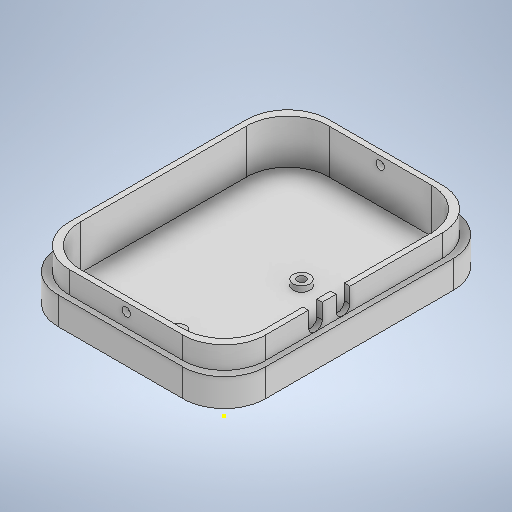
# Autodesk Inventor part: reduced_tortoise_3_base
Saved by Autodesk Inventor 2025.1 (Build 291241000, 241)
## iProperties
Created: 2025-04-15
Part Number: reduced_tortoise_3_base
Material: Generic
Document SubType Name: Modeling
Designer: Ian Ching
Density: 1 g/cm^3
Appearance: Default
Author: Ian Ching
Autodesk Inventor part; units mm, degrees
ref_plane "YZ Plane" through (0, 0, 0) normal (1, 0, 0) x (0, 1, 0)
ref_plane "XZ Plane" through (0, 0, 0) normal (0, 1, 0) x (-1, 0, 0)
ref_plane "XY Plane" through (0, 0, 0) normal (0, 0, 1) x (1, 0, 0)
sketch "Sketch1" plane through (0, 0, 0) normal (0, 1, 0) x (-1, 0, 0)
  line L0 (0, 0) -> (75, 0)
  line L1 (75, 0) -> (75, -98)
  line L2 (75, -98) -> (0, -98)
  line L3 (0, -98) -> (0, 0)
  dimension "d0" = 75
  dimension "d1" = 98
  constraints: 8 end point, 2 parallel, 1 horizontal, 1 perpendicular
  measures "d0" distance of L1.end L2.end
  measures "d1" distance of L0.end L1.end
extrude "Extrusion1" add sketch "Sketch1" along normal blind 2
sketch "Sketch2" plane through (0, 2, 0) normal (0, 1, 0) x (1, 0, 0)
  line L0 (-75, 0) -> (0, 0)
  line L1 (0, 0) -> (0, 98)
  line L2 (0, 98) -> (-75, 98)
  line L3 (-75, 98) -> (-75, 0)
  line L4 (-73, 2) -> (-2, 2)
  line L5 (-2, 2) -> (-2, 96)
  line L6 (-2, 96) -> (-73, 96)
  line L7 (-73, 96) -> (-73, 2)
  line L8 (-37.5, 2) -> (-37.5, 96)
  line L9 (-37.5, 0) -> (-37.5, 98)
  line L10 (-75, 0) -> (0, 0) projected
  line L11 (-37.5, 0) -> (-37.5, 98)
  line L12 (0, 98) -> (-75, 98) projected
  point P0 (-37.5, 49)
  dimension "d4" = 75
  dimension "d5" = 98
  dimension "d6" = 71
  dimension "d7" = 94
  constraints: 22 end point, 9 midpoint, 4 parallel, 2 horizontal, 2 perpendicular
  measures "d4" distance of L2.end L1.end
  measures "d5" distance of L1.end L0.end
  measures "d6" distance of L6.end L5.end
  measures "d7" distance of L5.end L4.end
extrude "Extrusion2" add sketch "Sketch2" along normal blind 8 contours L3 L2 L9 L6 L7 L4 L0 | L9 L4 L5 L6 L2 L1 L0
sketch "Sketch5" plane through (0, 2, 0) normal (0, 1, 0) x (1, 0, 0)
  line L0 (-2, 2) -> (-73, 2) projected
  line L1 (-73, 96) -> (-2, 96) projected
  line L2 (-2, 2) -> (-73, 2)
  line L3 (-73, 2) -> (-73, 96)
  line L4 (-73, 96) -> (-2, 96)
  line L5 (-2, 96) -> (-2, 2)
  line L6 (-4, 4) -> (-71, 4)
  line L7 (-71, 4) -> (-71, 94)
  line L8 (-71, 94) -> (-4, 94)
  line L9 (-4, 94) -> (-4, 4)
  line L10 (-37.5, 4) -> (-37.5, 94)
  line L11 (-37.5, 2) -> (-37.5, 96)
  point P0 (0, 0)
  point P1 (-37.5, 49)
  dimension "d11" = 67
  dimension "d12" = 90
  constraints: 20 end point, 6 midpoint, 4 parallel, 2 horizontal, 2 perpendicular
  measures "d11" distance of L7.end L8.end
  measures "d12" distance of L6.end L7.end
extrude "Extrusion3" add sketch "Sketch5" along normal blind 16 contours L0 L11 L6 L9 L8 L1 L5 | L0 L3 L1 L11 L8 L7 L6
fillet "Fillet2" radius 15 12 edges at (0, 5, 0) (-2, 14, -2) (0, 5, -98) (-2, 14, -96) (-75, 5, -98) (-73, 14, -96) (-71, 10, -4) (-75, 5, 0) (-73, 14, -2) (-4, 10, -4) (-71, 10, -94) (-4, 10, -94)
sketch "Sketch6" plane through (0, 2, 0) normal (0, 1, 0) x (1, 0, 0)
  line L0 (-18.5, 14) -> (-56.5, 14)
  line L1 (-56.5, 14) -> (-56.5, 68)
  line L2 (-56.5, 68) -> (-18.5, 68)
  line L3 (-18.5, 68) -> (-18.5, 14)
  line L4 (-18.5, 14) -> (-33.5, 14)
  line L5 (-33.5, 14) -> (-33.5, 16.5)
  line L6 (-33.5, 16.5) -> (-18.5, 16.5)
  line L7 (-18.5, 16.5) -> (-18.5, 14)
  line L8 (-18.5, 14) -> (-27, 14)
  line L9 (-27, 14) -> (-27, 55)
  line L10 (-27, 55) -> (-18.5, 55)
  line L11 (-18.5, 55) -> (-18.5, 14)
  circle A0 centre (-33.5, 16.5) radius 3
  circle A1 centre (-27, 55) radius 3
  line L12 (-19, 4) -> (-56, 4) projected
  line L13 (-37.5, 4) -> (-37.5, 94)
  line L14 (-19, 94) -> (-56, 94) projected
  line L15 (-37.5, 4) -> (-39.5, 4)
  line L16 (-39.5, 4) -> (-39.5, 14)
  line L17 (-39.5, 14) -> (-37.5, 14)
  line L18 (-37.5, 14) -> (-37.5, 4)
  point P0 (0, 0)
  dimension "d16" = 38
  dimension "d17" = 54
  dimension "d18" = 15
  dimension "d19" = 2.5
  dimension "d20" = 8.5
  dimension "d21" = 41
  dimension "d22" = 6
  dimension "d23" = 6
  dimension "d24" = 2
  dimension "d25" = 10
  constraints: 34 end point, 8 parallel, 4 horizontal, 4 perpendicular, 3 midpoint, 2 centre point, 2 coincident
  measures "d16" distance of L1.end L2.end
  measures "d17" distance of L0.end L1.end
  measures "d18" distance of L5.end L6.end
  measures "d19" distance of L4.end L5.end
  measures "d20" distance of L9.end L10.end
  measures "d21" distance of L8.end L9.end
  measures "d22" diameter of A0
  measures "d23" diameter of A1
  measures "d24" distance of L17.end L16.end
  measures "d25" distance of L16.end L15.end
extrude "Extrusion4" add sketch "Sketch6" along normal blind 2 contours A0 L0 | L0 L5 L6 A0 | L0 A0 L6 L5 | A1 L10 L9 | L9 L10 A1
sketch "Sketch7" plane through (-33.5, 4, -16.5) normal (0, 1, 0) x (1, 0, 0)
  circle A0 centre (0, 0) radius 3 projected
  circle A1 centre (0, 0) radius 1.5
  circle A2 centre (6.5, 38.5) radius 3 projected
  circle A3 centre (6.5, 38.5) radius 1.5
  point P0 (33.5, -16.5)
  dimension "d28" = 3
  dimension "d29" = 3
  constraints: 2 centre point, 2 coincident
  measures "d28" diameter of A1
  measures "d29" diameter of A3
extrude "Extrusion5" cut sketch "Sketch7" against normal blind 3 contours A1 | A3
sketch "Sketch8" plane through (-17, 18, -96) normal (0, 0, -1) x (-1, 0, 0)
  line L0 (41, -8) -> (41, 0) projected
  line L1 (41, -8) -> (0, -8)
  line L2 (0, -8) -> (0, -3)
  line L3 (0, -3) -> (41, -3)
  line L4 (41, -3) -> (41, -8)
  circle A0 centre (20.5, -3) radius 1.5
  point P0 (-17, -18)
  dimension "d32" = 41
  dimension "d33" = 5
  dimension "d34" = 3
  constraints: 8 end point, 2 parallel, 1 centre point, 1 horizontal, 1 midpoint, 1 perpendicular
  measures "d32" distance of L2.end L3.end
  measures "d33" distance of L1.end L2.end
  measures "d34" diameter of A0
extrude "Extrusion6" cut sketch "Sketch8" against normal blind 100 contours A0 L3 | L3 A0
sketch "Sketch9" plane through (0, 2, 0) normal (0, 1, 0) x (1, 0, 0)
  point P0 (0, 0)
sketch "Sketch10" plane through (-2, 10, -81) normal (1, 0, 0) x (0, 0, -1)
  line L0 (-66, -10) -> (-66, 0) projected
  line L1 (-66, 0) -> (-46, 0)
  line L2 (-46, 0) -> (-46, 2.5)
  line L3 (-46, 2.5) -> (-66, 2.5)
  line L4 (-66, 2.5) -> (-66, 0)
  line L5 (-66, 0) -> (-36, 0)
  line L6 (-36, 0) -> (-36, 2.5)
  line L7 (-36, 2.5) -> (-66, 2.5)
  line L8 (-66, 2.5) -> (-66, 0)
  circle A0 centre (-46, 2.5) radius 2.5
  circle A1 centre (-36, 2.5) radius 2.5
  line L9 (-48.5, 2.5) -> (-48.5, 8)
  line L10 (-2, 8) -> (-62, 8) projected
  line L11 (-43.5, 2.5) -> (-43.5, 8)
  line L12 (-38.5, 2.5) -> (-38.5, 8)
  line L13 (-33.5, 2.5) -> (-33.5, 8)
  point P0 (-81, -10)
  dimension "d37" = 20
  dimension "d38" = 2.5
  dimension "d39" = 30
  dimension "d40" = 2.5
  dimension "d41" = 5
  dimension "d42" = 5
  constraints: 24 end point, 9 point on line, 5 parallel, 4 point on circle, 3 tangent, 2 centre point, 2 coincident, 2 horizontal, 2 perpendicular, 1 vertical
  measures "d37" distance of L3.end L2.end
  measures "d38" distance of L2.end L1.end
  measures "d39" distance of L7.end L6.end
  measures "d40" distance of L6.end L5.end
  measures "d41" diameter of A0
  measures "d42" diameter of A1
extrude "Extrusion7" cut sketch "Sketch10" against normal blind 5 contours A0 L3 L2 | L2 L7 A0 | L3 A0 L7 | A1 L7 L6 | L6 L7 A1 | L9 L10 L11 A0 | L12 L10 L13 A1
body "Solid1"
